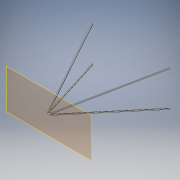
# Autodesk Inventor part: rearCrumpTail
Saved by Autodesk Inventor 2018 (Build 220112000, 112)
## iProperties
Created: 2018-03-26
Part Number: rearCrumpTail
Material: Generic
Document SubType Name: Modeling
Designer: rochee19
Density: 1 g/cm^3
Appearance: Default
Author: rochee19
Autodesk Inventor part; units mm, degrees
ref_plane "YZ Plane" through (0, 0, 0) normal (1, 0, 0) x (0, 1, 0)
ref_plane "XZ Plane" through (0, 0, 0) normal (0, 1, 0) x (-1, 0, 0)
ref_plane "XY Plane" through (0, 0, 0) normal (0, 0, 1) x (1, 0, 0)
sketch "Sketch1" plane through (0, 0, 0) normal (0, 0, 1) x (1, 0, 0)
  line L0 (-482.6, -222.25) -> (482.6, -222.25)
  line L1 (482.6, -222.25) -> (482.6, 222.25)
  line L2 (482.6, 222.25) -> (-482.6, 222.25)
  line L3 (-482.6, 222.25) -> (-482.6, -222.25)
  line L4 (-482.6, -222.25) -> (482.6, 222.25) construction
  line L5 (482.6, -222.25) -> (-482.6, 222.25) construction
  point P0 (0, 0)
  dimension "d0" = 965.2
  dimension "d1" = 444.5
  constraints: 12 end point, 2 midpoint, 2 parallel, 1 horizontal, 1 perpendicular
  measures "d0" distance of L2.end L1.end
  measures "d1" distance of L1.end L0.end
extrude "Extrusion1" add sketch "Sketch1" along normal blind 2.54
ref_plane "Work Plane1" through (0, 0, 1018.54) normal (0, 0, 1) x (1, 0, 0)
sketch "Sketch2" plane through (0, 0, 1018.54) normal (0, 0, 1) x (1, 0, 0)
  line L0 (-19.05, -9.525) -> (19.05, -9.525)
  line L1 (19.05, -9.525) -> (19.05, 9.525)
  line L2 (19.05, 9.525) -> (-19.05, 9.525)
  line L3 (-19.05, 9.525) -> (-19.05, -9.525)
  line L4 (-19.05, -9.525) -> (19.05, 9.525) construction
  line L5 (19.05, -9.525) -> (-19.05, 9.525) construction
  point P0 (0, 0)
  dimension "d5" = 38.1
  dimension "d6" = 19.05
  constraints: 12 end point, 2 midpoint, 2 parallel, 1 horizontal, 1 perpendicular
  measures "d5" distance of L2.end L1.end
  measures "d6" distance of L1.end L0.end
loft "Loft1" add profiles "Sketch2" section 1 edges at (0, -222.25, 2.54) (482.6, 0, 2.54) (0, 222.25, 2.54) (-482.6, 0, 2.54)
sketch "Sketch3" plane through (0, 0, 0) normal (0, 0, -1) x (-1, 0, 0)
  line L0 (-482.6, 222.25) -> (482.6, 222.25) projected
  line L1 (-482.6, -222.25) -> (482.6, -222.25)
  line L2 (482.6, -222.25) -> (482.6, 222.25)
  line L3 (482.6, 222.25) -> (-482.6, 222.25)
  line L4 (-482.6, 222.25) -> (-482.6, -222.25)
  line L5 (-482.6, -222.25) -> (482.6, 222.25) construction
  line L6 (482.6, -222.25) -> (-482.6, 222.25) construction
  point P0 (0, 0)
  constraints: 12 end point, 2 midpoint, 2 parallel, 1 horizontal, 1 perpendicular
extrude "Extrusion2" cut sketch "Sketch3" against normal blind 2.54
shell "Shell1" thickness 8.4667 removed faces 1 at (160.8667, 74.0833, 2.54)
sketch "Sketch4" plane through (482.6, -222.25, 2.54) normal (0.9097814, 0, 0.4150878) x (0.4150878, 0, -0.9097814)
  line L0 (0, 0) -> (0, 444.5) projected
  line L1 (0, 444.5) -> (-1116.7518, 231.775) projected
  line L2 (0, 444.5) -> (-1116.7518, 231.775)
  line L3 (-1116.7518, 231.775) -> (-1115.1675, 223.4579)
  line L4 (-1115.1675, 223.4579) -> (1.5843, 436.1829)
  line L5 (1.5843, 436.1829) -> (0, 444.5)
  line L6 (-1116.7518, 212.725) -> (-1132.5667, 212.725) projected
  line L7 (0, 0) -> (-1116.7518, 212.725)
  line L8 (-1116.7518, 212.725) -> (-1115.1675, 221.0421)
  line L9 (-1115.1675, 221.0421) -> (1.5843, 8.3171)
  line L10 (1.5843, 8.3171) -> (0, 0)
  line L11 (0, 435.8811) -> (0, 8.6189)
  line L12 (0, 8.6189) -> (-1115.1675, 221.0421)
  line L13 (-1115.1675, 221.0421) -> (-1115.1675, 223.4579)
  line L14 (-1115.1675, 223.4579) -> (0, 435.8811)
  line L15 (0, 435.8811) -> (0, 8.6189)
  point P0 (-198.0105, 222.25)
  dimension "d14" = 8.4667
  dimension "d15" = 8.4667
  constraints: 26 end point, 5 parallel, 4 point on line, 2 collinear, 2 perpendicular, 1 vertical
  measures "d14" distance of L3.end L1.end
  measures "d15" distance of L6.start L8.end
extrude "Extrusion3" cut sketch "Sketch4" against normal blind 8.4667 contours L9 L13 L4 L0
sketch "Sketch5" plane through (-482.6, -222.25, 2.54) normal (-0.9097814, 0, 0.4150878) x (0.4150878, 0, 0.9097814)
  line L0 (0, 444.5) -> (1116.7518, 231.775) projected
  line L1 (0, 444.5) -> (0, 0) projected
  line L2 (1116.7518, 231.775) -> (0, 444.5)
  line L3 (0, 0) -> (1116.7518, 212.725) projected
  line L4 (1116.7518, 212.725) -> (0, 0)
  line L5 (0, 0) -> (-1.5843, 8.3171)
  line L6 (-1.5843, 8.3171) -> (1115.1675, 221.0421)
  line L7 (1115.1675, 221.0421) -> (1116.7518, 212.725)
  line L8 (400.6427, 444.5) -> (0, 444.5) projected
  line L9 (1116.7518, 231.775) -> (0, 444.5)
  line L10 (0, 444.5) -> (-1.5843, 436.1829)
  line L11 (-1.5843, 436.1829) -> (1115.1675, 223.4579)
  line L12 (1115.1675, 223.4579) -> (1116.7518, 231.775)
  line L13 (0, 8.6189) -> (0, 435.8811)
  line L14 (0, 435.8811) -> (1115.1675, 223.4579)
  line L15 (1116.7518, 212.725) -> (1116.7518, 231.775) projected
  line L16 (1115.1675, 223.4579) -> (1115.1675, 221.0421)
  line L17 (1115.1675, 221.0421) -> (0, 8.6189)
  point P0 (198.0105, 222.25)
  dimension "d18" = 8.4667
  dimension "d19" = 8.4667
  constraints: 26 end point, 4 parallel, 4 point on line, 3 perpendicular, 2 collinear
  measures "d18" distance of L1.end L5.end
  measures "d19" distance of L10.end L0.start
extrude "Extrusion4" cut sketch "Sketch5" against normal blind 8.4667 contours L11 L16 L6 L1
sketch "Sketch6" plane through (-19.05, 9.525, 1018.54) normal (0, 0.9787764, 0.2049313) x (1, 0, 0)
  line L0 (0, 0) -> (38.1, 0) projected
  line L1 (501.65, 1038.0308) -> (-463.55, 1038.0308) projected
  line L2 (38.1, 0) -> (501.65, 1038.0308)
  line L3 (501.65, 1038.0308) -> (493.9192, 1041.4831)
  line L4 (493.9192, 1041.4831) -> (30.3692, 3.4523)
  line L5 (30.3692, 3.4523) -> (38.1, 0)
  line L6 (0, -3.9039) -> (0, 0) projected
  line L7 (-463.55, 1038.0308) -> (-463.55, 1036.2645) projected
  line L8 (0, 0) -> (-463.55, 1038.0308)
  line L9 (-463.55, 1038.0308) -> (-455.8192, 1041.4831)
  line L10 (-455.8192, 1041.4831) -> (7.7308, 3.4523)
  line L11 (7.7308, 3.4523) -> (0, 0)
  line L12 (492.3775, 1038.0308) -> (-454.2775, 1038.0308)
  line L13 (-454.2775, 1038.0308) -> (7.7308, 3.4523)
  line L14 (30.3692, 3.4523) -> (7.7308, 3.4523)
  line L15 (30.3692, 3.4523) -> (492.3775, 1038.0308)
  point P0 (19.05, 994.9709)
  dimension "d22" = 8.4667
  dimension "d23" = 8.4667
  constraints: 24 end point, 4 parallel, 4 point on line, 2 perpendicular, 1 collinear
  measures "d22" distance of L3.end L1.start
  measures "d23" distance of L1.end L9.end
extrude "Extrusion5" cut sketch "Sketch6" against normal blind 8.4667 contours L10 L1 L4 L14
sketch "Sketch7" plane through (-19.05, -9.525, 1018.54) normal (0, -0.9787764, 0.2049313) x (1, 0, 0)
  line L0 (-463.55, -1038.0308) -> (501.65, -1038.0308) projected
  line L1 (-0.6576, 0.2937) -> (7.0452, -3.1462) projected
  line L2 (-463.55, -1038.0308) -> (0, 0)
  line L3 (0, 0) -> (7.7308, -3.4523)
  line L4 (7.7308, -3.4523) -> (-455.8192, -1041.4831)
  line L5 (-455.8192, -1041.4831) -> (-463.55, -1038.0308)
  line L6 (501.65, -1038.0308) -> (501.65, -1036.2645) projected
  line L7 (38.1, 0) -> (0, 0) projected
  line L8 (501.65, -1038.0308) -> (38.1, 0)
  line L9 (38.1, 0) -> (30.3692, -3.4523)
  line L10 (30.3692, -3.4523) -> (493.9192, -1041.4831)
  line L11 (493.9192, -1041.4831) -> (501.65, -1038.0308)
  line L12 (30.3692, 0.7416) -> (30.3692, -2.6549) projected
  line L13 (7.7308, -3.4523) -> (30.3692, -3.4523)
  line L14 (30.3692, -3.4523) -> (492.3775, -1038.0308)
  line L15 (492.3775, -1038.0308) -> (-454.2775, -1038.0308)
  line L16 (-454.2775, -1038.0308) -> (7.7308, -3.4523)
  point P0 (19.05, -994.9709)
  dimension "d26" = 8.4667
  dimension "d27" = 8.4667
  constraints: 24 end point, 5 point on line, 4 parallel, 2 perpendicular
  measures "d26" distance of L2.end L3.end
  measures "d27" distance of L9.end L7.start
extrude "Extrusion6" cut sketch "Sketch7" against normal blind 8.4667 contours L4 L13 L10 L0
body "Solid1"
